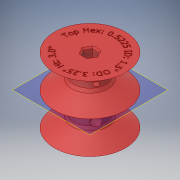
# Autodesk Inventor part: spoolV07
Saved by Autodesk Inventor 2019.4 (Build 234330000, 330)
## iProperties
Created: 2019-02-25
Part Number: spoolV07
Material: PC/ABS Plastic
Document SubType Name: Modeling
Designer: steele
Density: 0.357273 g/cm^3
Appearance: Smooth - Red
holeForString: 0.200 in
stringDiameter: 0.120 in
clearanceForString: 0.080 in
clearanceForHexShaft: 0.023 in
hexDiameter: 0.523 in
supportChannels: 0.150 in
spoolInteriorDiameter: 1.500 in
spoolInteriroRadius: 0.750 in
spoolExteriorDiameter: 3.250 in
spoolExteriorRadius: 1.625 in
spoolFiletRadius: 0.075 in
holeCenter: 0.575 in
hexHoleChamfer: 0.063 in
stringHoleCenterFromHexShaft: 0.361 in
textCircleDiameter: 2.438 in
textHeight: 0.240 in
textDepth: 0.050 in
stringHoleChamfer: 0.188 in
spoolTotalHeight: 3.000 in
spaceHeight: 0.250 in
spacerDiameter: 0.950 in
spoolHeightWithoutSpacer: 2.750 in
Author: steele
Autodesk Inventor part; units mm, degrees
(part 1 of 2)
ref_plane "XZ Plane" through (0, 0, 0) normal (0, 1, 0) x (-1, 0, 0)
ref_plane "XY Plane" through (0, 0, 0) normal (0, 0, 1) x (1, 0, 0)
sketch "Sketch15" plane through (0, 0, 0) normal (0, 0, 1) x (1, 0, 0)
  line L0 (41.275, 0) -> (41.275, 76.2) construction
  line L1 (0, 0) -> (41.275, 0)
  line L2 (0, 76.2) -> (41.275, 76.2)
  line L3 (19.05, 0) -> (19.05, 76.2) construction
  line L4 (0, 76.2) -> (0, 0)
  line L5 (19.05, 19.05) -> (41.275, 19.05) construction
  line L6 (41.275, 0) -> (19.05, 12.8316)
  line L7 (41.275, 38.1) -> (19.05, 25.2684)
  line L8 (19.05, 25.2684) -> (41.275, 25.2684) construction
  line L9 (19.05, 25.2684) -> (19.05, 12.8316)
  line L10 (41.275, 38.1) -> (19.05, 50.9316)
  line L11 (19.05, 50.9316) -> (19.05, 63.3684)
  line L12 (19.05, 63.3684) -> (41.275, 76.2)
  line L13 (41.275, 38.1) -> (19.05, 38.1) construction
  line L14 (19.05, 63.3684) -> (41.275, 63.3684) construction
  dimension "d85" = 41.275
  dimension "d86" = 76.2
  dimension "d87" = 19.05
  dimension "d88" = 41.275
  dimension "d89" = 38.1
  dimension "centerLineForSpool" = 19.05
  dimension "d93" = 30
  dimension "d94" = 30
  dimension "d95" = 30
  dimension "d96" = 30
  constraints: 30 end point, 10 point on line, 3 horizontal, 2 midpoint, 2 perpendicular, 1 collinear, 1 parallel, 1 vertical
  measures "d85" distance from line of L1.start L0
  measures "d86" distance of L0.start L0.end
  measures "d87" distance from line of L3 L1.start
  measures "d88" distance of L2.start L0.end
  measures "d89" distance from line of L7.start L1
  measures "centerLineForSpool" distance from line of L5.start L1
  measures "d93" angle of L6 L1
  measures "d94" angle of L7 L8
  measures "d95" angle of L10 L13
  measures "d96" angle of L12 L14
revolve "Revolution2" add sketch "Sketch15" angle 360 about axis through (0, 76.2, 0) along (0, -1, 0)
sketch "Sketch16" plane through (0, 0, 0) normal (0, -1, 0) x (1, 0, 0)
  line L0 (-7.6623, 0) -> (-3.8312, 6.6357)
  line L1 (-3.8312, 6.6357) -> (3.8312, 6.6357)
  line L2 (3.8312, 6.6357) -> (7.6623, 0)
  line L3 (7.6623, 0) -> (3.8312, -6.6358)
  line L4 (3.8312, -6.6358) -> (-3.8312, -6.6358)
  line L5 (-3.8312, -6.6358) -> (-7.6623, 0)
  point P0 (0, 0)
  point P1 (0, 0)
  dimension "d103" = 13.2715
  constraints: 12 end point, 1 coincident, 1 horizontal, 13 other
  measures "d103" distance between parallel lines of L1 L4
extrude "Extrusion11" cut sketch "Sketch16" against normal through all
sketch "Sketch17" plane through (0, 0, 0) normal (1, 0, 0) x (0, 1, 0)
  circle A0 centre (57.15, 9.1757) radius 2.54
  circle A1 centre (19.05, 9.1757) radius 2.54
  line L0 (0, 41.275) -> (0, -41.275) projected
  line L1 (76.2, 41.275) -> (76.2, -41.275) projected
  line L2 (0, 6.6357) -> (76.2, 6.6357) projected
  point P0 (0, 0)
  dimension "d110" = 19.05
  dimension "d111" = 19.05
  dimension "d112" = 5.08
  constraints: 2 centre point, 2 tangent, 1 equal radius
  measures "d110" distance from line of A1.centre L0
  measures "d111" distance from line of A0.centre L1
  measures "d112" diameter of A0
extrude "Extrusion13" cut sketch "Sketch17" along normal through all both and the other way through all
ref_plane "Work Plane4" through (-19.05, 0, 0) normal (1, 0, 0) x (0, 1, 0)
sketch "Sketch22" plane through (-19.05, 0, 0) normal (1, 0, 0) x (0, 1, 0)
  spline S0 degree 8 poles (59.69, 9.1757) (59.69, 9.4517) (59.6557, 9.7212) (59.59, 9.9804) (59.4956, 10.2261) (59.3755, 10.4557) (59.2323, 10.6669) (59.0691, 10.858) (58.7144, 11.191) (58.5225, 11.336) (58.3154, 11.4599) (58.0958, 11.5609) (57.8667, 11.6378) (57.6308, 11.6896) (57.3909, 11.7157) (56.8686, 11.7157) (56.5893, 11.6801) (56.3163, 11.6098) (56.0539, 11.5059) (55.8062, 11.37) (55.5775, 11.2041) (55.3719, 11.0111) (55.0147, 10.5794) (54.8595, 10.3366) (54.7333, 10.0693) (54.6415, 9.7817) (54.5882, 9.479) (54.5771, 9.1672) (54.6105, 8.8531) (54.8032, 8.1024) (55.0034, 7.6991) (55.2751, 7.3483) (55.6037, 7.0608) (55.9729, 6.8444) (56.3656, 6.703) (56.7635, 6.6357) (57.4276, 6.6357) (57.7065, 6.6704) (57.9827, 6.7403) (58.2517, 6.8459) (58.509, 6.9871) (58.7494, 7.1637) (58.9676, 7.3748) (59.2832, 7.7816) (59.3962, 7.9584) (59.4932, 8.1474) (59.5721, 8.3459) (59.6315, 8.5511) (59.6708, 8.76) (59.69, 8.9692) (59.69, 9.1757) knots 0 0 0 0 0 0 0 0 0 0.129052 0.129052 0.129052 0.129052 0.129052 0.129052 0.129052 0.253777 0.253777 0.253777 0.253777 0.253777 0.253777 0.253777 0.399469 0.399469 0.399469 0.399469 0.399469 0.399469 0.399469 0.544533 0.544533 0.544533 0.544533 0.544533 0.544533 0.544533 0.751894 0.751894 0.751894 0.751894 0.751894 0.751894 0.751894 0.900801 0.900801 0.900801 0.900801 0.900801 0.900801 0.900801 1 1 1 1 1 1 1 1 1 projected
  circle A0 centre (57.15, 9.1757) radius 4.7625
  circle A1 centre (57.15, 9.1757) radius 2.54 construction
  line L0 (57.15, 6.6357) -> (76.2, 6.6357) construction
  line L1 (76.2, 41.275) -> (76.2, -41.275) construction
  point P0 (0, 0)
  dimension "d121" = 19.05
  dimension "d122" = 5.08
  dimension "d125" = 9.525
  constraints: 2 centre point, 1 concentric, 1 tangent, 1 vertical alignment
  measures "d121" distance from line of A1.centre L1
  measures "d122" diameter of A1
  measures "d125" diameter of A0
extrude "Extrusion16" cut sketch "Sketch22" along normal blind 11.1125
ref_plane "Work Plane5" through (19.05, 0, 0) normal (1, 0, 0) x (0, 1, 0)
sketch "Sketch23" plane through (19.05, 0, 0) normal (1, 0, 0) x (0, 1, 0)
  line L0 (19.05, 6.6357) -> (57.15, 6.6357) projected
  circle A0 centre (19.05, 9.1757) radius 2.54 construction
  line L1 (0, 41.275) -> (0, -41.275) projected
  circle A1 centre (19.05, 9.1757) radius 4.7625
  point P0 (0, 0)
  dimension "d127" = 5.08
  dimension "d128" = 19.05
  dimension "d129" = 9.525
  constraints: 2 centre point, 1 coincident, 1 tangent
  measures "d127" diameter of A0
  measures "d128" distance from line of A0.centre L1
  measures "d129" diameter of A1
extrude "Extrusion17" cut sketch "Sketch23" against normal blind 11.1125
chamfer "Chamfer10" distance 1.5875 angle 45 12 edges at (0, 76.2, -6.6358) (5.7467, 76.2, -3.3179) (5.7467, 76.2, 3.3179) (0, 76.2, 6.6357) (-5.7467, 76.2, 3.3179) (-5.7467, 76.2, -3.3179) (-5.7467, 0, -3.3179) (-5.7467, 0, 3.3179) (0, 0, 6.6357) (5.7467, 0, 3.3179) (5.7467, 0, -3.3179) (0, 0, -6.6358)
chamfer "Chamfer12" distance 2.3813 angle 45 4 edges at (-19.05, 63.3684, 0) (-19.05, 50.9316, 0) (-19.05, 25.2684, 0) (-19.05, 12.8316, 0)
ref_plane "Work Plane6" through (0, 38.1, 0) normal (0, -1, 0) x (1, 0, 0)
sketch "Sketch24" plane through (0, 76.2, 0) normal (0, 1, 0) x (1, 0, 0)
  circle A0 centre (0, 0) radius 28.575 construction
  line L0 (-28.5056, 2.0328) -> (-33.8607, 2.492)
  line L1 (-33.8607, 2.492) -> (-34.0354, 0.4543)
  line L2 (-34.0354, 0.4543) -> (-34.754, 0.5159)
  line L3 (-34.754, 0.5159) -> (-34.3353, 5.3985)
  line L4 (-34.3353, 5.3985) -> (-33.6167, 5.3369)
  line L5 (-33.6167, 5.3369) -> (-33.7914, 3.2992)
  line L6 (-33.7914, 3.2992) -> (-28.4363, 2.84)
  line L7 (-28.4363, 2.84) -> (-28.5056, 2.0328)
  spline S0 degree 2 poles (-29.3924, 9.63) (-28.2725, 9.3434) (-27.3277, 7.9543) (-27.5579, 7.0546) knots 0 0 0 1 2 2 2
  spline S1 degree 2 poles (-27.5579, 7.0546) (-27.7943, 6.1309) (-29.3236, 5.3953) (-30.4052, 5.6721) knots 0 0 0 1 2 2 2
  spline S2 degree 2 poles (-30.4052, 5.6721) (-31.5155, 5.9562) (-32.4663, 7.3621) (-32.2385, 8.2523) knots 0 0 0 1 2 2 2
  spline S3 degree 2 poles (-32.2385, 8.2523) (-32.0082, 9.152) (-30.5075, 9.9153) (-29.3924, 9.63) knots 0 0 0 1 2 2 2
  spline S4 degree 2 poles (-29.5896, 8.8595) (-30.451, 9.0799) (-31.449, 8.6673) (-31.5972, 8.0882) knots 0 0 0 1 2 2 2
  spline S5 degree 2 poles (-31.5972, 8.0882) (-31.7454, 7.5091) (-31.0695, 6.6631) (-30.208, 6.4426) knots 0 0 0 1 2 2 2
  spline S6 degree 2 poles (-30.208, 6.4426) (-29.3705, 6.2283) (-28.3474, 6.6396) (-28.1992, 7.2187) knots 0 0 0 1 2 2 2
  spline S7 degree 2 poles (-28.1992, 7.2187) (-28.0523, 7.793) (-28.7377, 8.6415) (-29.5896, 8.8595) knots 0 0 0 1 2 2 2
  spline S8 degree 2 poles (-27.5782, 14.278) (-26.5275, 13.8203) (-25.7227, 12.2788) (-26.0561, 11.5134) knots 0 0 0 1 2 2 2
  spline S9 degree 2 poles (-26.0561, 11.5134) (-26.1923, 11.2009) (-26.5463, 10.784) (-26.8043, 10.6) knots 0 0 0 1 2 2 2
  line L8 (-26.8043, 10.6) -> (-25.0471, 9.8344)
  line L9 (-25.0471, 9.8344) -> (-25.3549, 9.1279)
  line L10 (-25.3549, 9.1279) -> (-31.093, 11.6278)
  line L11 (-31.093, 11.6278) -> (-30.7852, 12.3343)
  line L12 (-30.7852, 12.3343) -> (-30.3459, 12.1429)
  spline S10 degree 2 poles (-30.3459, 12.1429) (-30.4715, 12.5102) (-30.5083, 13.2914) (-30.3446, 13.6673) knots 0 0 0 1 2 2 2
  spline S11 degree 2 poles (-30.3446, 13.6673) (-30.0308, 14.3874) (-28.5384, 14.6963) (-27.5782, 14.278) knots 0 0 0 1 2 2 2
  spline S12 degree 2 poles (-27.8144, 13.5133) (-28.5345, 13.8271) (-29.5263, 13.7149) (-29.7493, 13.2032) knots 0 0 0 1 2 2 2
  spline S13 degree 2 poles (-29.7493, 13.2032) (-29.8795, 12.9043) (-29.8569, 12.2263) (-29.7571, 11.8864) knots 0 0 0 1 2 2 2
  line L13 (-29.7571, 11.8864) -> (-27.3749, 10.8486)
  spline S14 degree 2 poles (-27.3749, 10.8486) (-27.1232, 11.0676) (-26.852, 11.4182) (-26.7415, 11.6718) knots 0 0 0 1 2 2 2
  spline S15 degree 2 poles (-26.7415, 11.6718) (-26.5027, 12.2198) (-27.0445, 13.1779) (-27.8144, 13.5133) knots 0 0 0 1 2 2 2
  line L14 (-20.7867, 19.7317) -> (-21.2974, 19.1028)
  line L15 (-21.2974, 19.1028) -> (-23.6136, 20.9838)
  line L16 (-23.6136, 20.9838) -> (-25.3825, 18.8057)
  line L17 (-25.3825, 18.8057) -> (-23.0663, 16.9247)
  line L18 (-23.0663, 16.9247) -> (-23.577, 16.2958)
  line L19 (-23.577, 16.2958) -> (-28.3092, 20.1387)
  line L20 (-28.3092, 20.1387) -> (-27.7984, 20.7676)
  line L21 (-27.7984, 20.7676) -> (-25.9424, 19.2603)
  line L22 (-25.9424, 19.2603) -> (-24.1735, 21.4385)
  line L23 (-24.1735, 21.4385) -> (-26.0296, 22.9458)
  line L24 (-26.0296, 22.9458) -> (-25.5188, 23.5747)
  line L25 (-25.5188, 23.5747) -> (-20.7867, 19.7317)
  spline S16 degree 2 poles (-18.3661, 21.758) (-19.1957, 21.0407) (-20.912, 21.1828) (-21.6552, 22.0423) knots 0 0 0 1 2 2 2
  spline S17 degree 2 poles (-21.6552, 22.0423) (-22.3854, 22.8868) (-22.3657, 24.654) (-21.652, 25.2712) knots 0 0 0 1 2 2 2
  spline S18 degree 2 poles (-21.652, 25.2712) (-21.3306, 25.5491) (-20.6721, 25.792) (-20.3177, 25.7522) knots 0 0 0 1 2 2 2
  spline S19 degree 2 poles (-20.3177, 25.7522) (-19.9596, 25.7157) (-19.2672, 25.3152) (-18.9086, 24.9005) knots 0 0 0 1 2 2 2
  line L26 (-18.9086, 24.9005) -> (-18.6339, 24.5828)
  line L27 (-18.6339, 24.5828) -> (-21.0292, 22.5117)
  spline S20 degree 2 poles (-21.0292, 22.5117) (-20.509, 21.9101) (-19.3511, 21.7945) (-18.813, 22.2598) knots 0 0 0 1 2 2 2
  spline S21 degree 2 poles (-18.813, 22.2598) (-18.6225, 22.4246) (-18.3268, 22.8304) (-18.2355, 23.0269) knots 0 0 0 1 2 2 2
  spline S22 degree 2 poles (-18.2355, 23.0269) (-18.1432, 23.2373) (-18.0396, 23.5555) (-18.0203, 23.6767) knots 0 0 0 1 2 2 2
  line L28 (-18.0203, 23.6767) -> (-17.9866, 23.7058)
  line L29 (-17.9866, 23.7058) -> (-17.4373, 23.0705)
  spline S23 degree 2 poles (-17.4373, 23.0705) (-17.5027, 22.9422) (-17.7057, 22.5577) (-17.7962, 22.4206) knots 0 0 0 1 2 2 2
  spline S24 degree 2 poles (-17.7962, 22.4206) (-17.9224, 22.2267) (-18.1569, 21.939) (-18.3661, 21.758) knots 0 0 0 1 2 2 2
  spline S25 degree 2 poles (-19.5864, 24.5364) (-19.7975, 24.7653) (-20.1919, 25.0251) (-20.3855, 25.0602) knots 0 0 0 1 2 2 2
  spline S26 degree 2 poles (-20.3855, 25.0602) (-20.5995, 25.1037) (-21.0366, 24.9673) (-21.2721, 24.7638) knots 0 0 0 1 2 2 2
  spline S27 degree 2 poles (-21.2721, 24.7638) (-21.5037, 24.5635) (-21.7093, 24.1441) (-21.7275, 23.8932) knots 0 0 0 1 2 2 2
  spline S28 degree 2 poles (-21.7275, 23.8932) (-21.7387, 23.6419) (-21.5857, 23.193) (-21.4137, 22.9564) knots 0 0 0 1 2 2 2
  line L30 (-21.4137, 22.9564) -> (-19.5864, 24.5364)
  line L31 (-13.5409, 25.2452) -> (-14.3386, 24.7412)
  line L32 (-14.3386, 24.7412) -> (-16.1964, 25.601)
  line L33 (-16.1964, 25.601) -> (-16.243, 23.5381)
  line L34 (-16.243, 23.5381) -> (-16.9823, 23.0711)
  line L35 (-16.9823, 23.0711) -> (-16.8526, 25.835)
  line L36 (-16.8526, 25.835) -> (-19.4129, 26.9464)
  line L37 (-19.4129, 26.9464) -> (-18.6152, 27.4503)
  line L38 (-18.6152, 27.4503) -> (-16.7694, 26.6005)
  line L39 (-16.7694, 26.6005) -> (-16.7233, 28.6455)
  line L40 (-16.7233, 28.6455) -> (-15.984, 29.1125)
  line L41 (-15.984, 29.1125) -> (-16.1106, 26.3623)
  line L42 (-16.1106, 26.3623) -> (-13.5409, 25.2452)
  line L43 (-13.1552, 29.157) -> (-14.0405, 28.7412)
  line L44 (-14.0405, 28.7412) -> (-14.5362, 29.7964)
  line L45 (-14.5362, 29.7964) -> (-13.6509, 30.2123)
  line L46 (-13.6509, 30.2123) -> (-13.1552, 29.157)
  line L47 (-11.706, 26.0718) -> (-12.5914, 25.6559)
  line L48 (-12.5914, 25.6559) -> (-13.087, 26.7112)
  line L49 (-13.087, 26.7112) -> (-12.2017, 27.127)
  line L50 (-12.2017, 27.127) -> (-11.706, 26.0718)
  spline S29 degree 2 poles (-4.8677, 31.307) (-4.5164, 29.705) (-5.1186, 28) (-6.0885, 27.7873) knots 0 0 0 1 2 2 2
  spline S30 degree 2 poles (-6.0885, 27.7873) (-7.0729, 27.5715) (-8.33, 28.899) (-8.6739, 30.4673) knots 0 0 0 1 2 2 2
  spline S31 degree 2 poles (-8.6739, 30.4673) (-9.0273, 32.0789) (-8.423, 33.7742) (-7.4483, 33.9879) knots 0 0 0 1 2 2 2
  spline S32 degree 2 poles (-7.4483, 33.9879) (-6.4687, 34.2028) (-5.2085, 32.8607) (-4.8677, 31.307) knots 0 0 0 1 2 2 2
  spline S33 degree 2 poles (-5.4928, 29.2683) (-5.4416, 29.5881) (-5.544, 30.5164) (-5.6784, 31.1292) knots 0 0 0 1 2 2 2
  spline S34 degree 2 poles (-5.6784, 31.1292) (-5.8128, 31.742) (-6.1072, 32.6232) (-6.2945, 32.9008) knots 0 0 0 1 2 2 2
  spline S35 degree 2 poles (-6.2945, 32.9008) (-6.4818, 33.1783) (-6.9704, 33.3999) (-7.3033, 33.3269) knots 0 0 0 1 2 2 2
  spline S36 degree 2 poles (-7.3033, 33.3269) (-7.6363, 33.2539) (-7.9969, 32.846) (-8.0536, 32.5049) knots 0 0 0 1 2 2 2
  spline S37 degree 2 poles (-8.0536, 32.5049) (-8.1076, 32.1744) (-7.9913, 31.2289) (-7.8632, 30.645) knots 0 0 0 1 2 2 2
  spline S38 degree 2 poles (-7.8632, 30.645) (-7.7257, 30.0177) (-7.4643, 29.195) (-7.2669, 28.8944) knots 0 0 0 1 2 2 2
  spline S39 degree 2 poles (-7.2669, 28.8944) (-7.0834, 28.611) (-6.5809, 28.3722) (-6.2335, 28.4484) knots 0 0 0 1 2 2 2
  spline S40 degree 2 poles (-6.2335, 28.4484) (-5.9054, 28.5204) (-5.5447, 28.9282) (-5.4928, 29.2683) knots 0 0 0 1 2 2 2
  line L51 (-2.1318, 28.4995) -> (-3.1058, 28.41)
  line L52 (-3.1058, 28.41) -> (-3.2125, 29.571)
  line L53 (-3.2125, 29.571) -> (-2.2384, 29.6604)
  line L54 (-2.2384, 29.6604) -> (-2.1318, 28.4995)
  spline S41 degree 2 poles (2.8482, 30.4347) (2.8338, 29.9953) (2.5279, 29.254) (2.2621, 28.9859) knots 0 0 0 1 2 2 2
  spline S42 degree 2 poles (2.2621, 28.9859) (1.9963, 28.7178) (1.2205, 28.4219) (0.7465, 28.4373) knots 0 0 0 1 2 2 2
  spline S43 degree 2 poles (0.7465, 28.4373) (0.312, 28.4515) (-0.5309, 28.6719) (-0.8369, 28.8351) knots 0 0 0 1 2 2 2
  line L55 (-0.8369, 28.8351) -> (-0.8087, 29.6991)
  line L56 (-0.8087, 29.6991) -> (-0.7495, 29.6972)
  spline S44 degree 2 poles (-0.7495, 29.6972) (-0.6579, 29.625) (-0.3132, 29.4358) (-0.1034, 29.3499) knots 0 0 0 1 2 2 2
  spline S45 degree 2 poles (-0.1034, 29.3499) (0.1358, 29.258) (0.5326, 29.1511) (0.7844, 29.1429) knots 0 0 0 1 2 2 2
  spline S46 degree 2 poles (0.7844, 29.1429) (1.0313, 29.1348) (1.5012, 29.2974) (1.6754, 29.4845) knots 0 0 0 1 2 2 2
  spline S47 degree 2 poles (1.6754, 29.4845) (1.8344, 29.6622) (2.0082, 30.1409) (2.0189, 30.4667) knots 0 0 0 1 2 2 2
  spline S48 degree 2 poles (2.0189, 30.4667) (2.0295, 30.7926) (1.8653, 31.2132) (1.702, 31.3569) knots 0 0 0 1 2 2 2
  spline S49 degree 2 poles (1.702, 31.3569) (1.5342, 31.5156) (1.0249, 31.6608) (0.7138, 31.6709) knots 0 0 0 1 2 2 2
  spline S50 degree 2 poles (0.7138, 31.6709) (0.3781, 31.6819) (-0.2919, 31.6) (-0.4957, 31.5622) knots 0 0 0 1 2 2 2
  line L57 (-0.4957, 31.5622) -> (-0.3931, 34.7024)
  line L58 (-0.3931, 34.7024) -> (2.9495, 34.5931)
  line L59 (2.9495, 34.5931) -> (2.9261, 33.8772)
  line L60 (2.9261, 33.8772) -> (0.3685, 33.9608)
  line L61 (0.3685, 33.9608) -> (0.3154, 32.3364)
  spline S51 degree 2 poles (0.3154, 32.3364) (0.4642, 32.3513) (0.7511, 32.3567) (0.8696, 32.3529) knots 0 0 0 1 2 2 2
  spline S52 degree 2 poles (0.8696, 32.3529) (1.3386, 32.3375) (1.9804, 32.1633) (2.2692, 31.9265) knots 0 0 0 1 2 2 2
  spline S53 degree 2 poles (2.2692, 31.9265) (2.563, 31.6896) (2.8663, 30.9877) (2.8482, 30.4347) knots 0 0 0 1 2 2 2
  line L62 (7.3458, 27.6811) -> (3.6558, 28.4)
  line L63 (3.6558, 28.4) -> (3.8211, 29.2486)
  spline S54 degree 2 poles (3.8211, 29.2486) (4.2915, 29.5445) (5.1345, 30.0999) (5.5467, 30.4072) knots 0 0 0 1 2 2 2
  spline S55 degree 2 poles (5.5467, 30.4072) (6.3768, 31.0255) (7.0519, 31.8301) (7.1455, 32.3102) knots 0 0 0 1 2 2 2
  spline S56 degree 2 poles (7.1455, 32.3102) (7.1946, 32.5623) (7.1131, 32.9707) (6.9961, 33.1194) knots 0 0 0 1 2 2 2
  spline S57 degree 2 poles (6.9961, 33.1194) (6.8791, 33.268) (6.5342, 33.461) (6.3112, 33.5044) knots 0 0 0 1 2 2 2
  spline S58 degree 2 poles (6.3112, 33.5044) (6.0978, 33.546) (5.6406, 33.5244) (5.4258, 33.4807) knots 0 0 0 1 2 2 2
  spline S59 degree 2 poles (5.4258, 33.4807) (5.2428, 33.4458) (4.8899, 33.3133) (4.7797, 33.2643) knots 0 0 0 1 2 2 2
  line L64 (4.7797, 33.2643) -> (4.736, 33.2728)
  line L65 (4.736, 33.2728) -> (4.9023, 34.1262)
  spline S60 degree 2 poles (4.9023, 34.1262) (5.1732, 34.1992) (6.1068, 34.264) (6.5044, 34.1865) knots 0 0 0 1 2 2 2
  spline S61 degree 2 poles (6.5044, 34.1865) (7.3433, 34.0231) (8.116, 32.9515) (7.9686, 32.1951) knots 0 0 0 1 2 2 2
  spline S62 degree 2 poles (7.9686, 32.1951) (7.8996, 31.8411) (7.6195, 31.2817) (7.4249, 31.0579) knots 0 0 0 1 2 2 2
  spline S63 degree 2 poles (7.4249, 31.0579) (7.2284, 30.8244) (6.7064, 30.3926) (6.4255, 30.1906) knots 0 0 0 1 2 2 2
  spline S64 degree 2 poles (6.4255, 30.1906) (5.967, 29.8522) (4.8689, 29.1501) (4.5425, 28.947) knots 0 0 0 1 2 2 2
  line L66 (4.5425, 28.947) -> (7.4809, 28.3745)
  line L67 (7.4809, 28.3745) -> (7.3458, 27.6811)
  line L68 (11.6554, 26.1602) -> (8.1268, 27.4569)
  line L69 (8.1268, 27.4569) -> (8.425, 28.2683)
  spline S65 degree 2 poles (8.425, 28.2683) (8.9364, 28.4857) (9.8571, 28.9) (10.3128, 29.1377) knots 0 0 0 1 2 2 2
  spline S66 degree 2 poles (10.3128, 29.1377) (11.2308, 29.6162) (12.0253, 30.3031) (12.194, 30.7622) knots 0 0 0 1 2 2 2
  spline S67 degree 2 poles (12.194, 30.7622) (12.2826, 31.0033) (12.2671, 31.4195) (12.1752, 31.5848) knots 0 0 0 1 2 2 2
  spline S68 degree 2 poles (12.1752, 31.5848) (12.0834, 31.7502) (11.7736, 31.9956) (11.5603, 32.074) knots 0 0 0 1 2 2 2
  spline S69 degree 2 poles (11.5603, 32.074) (11.3563, 32.1489) (10.9015, 32.2003) (10.6824, 32.1913) knots 0 0 0 1 2 2 2
  spline S70 degree 2 poles (10.6824, 32.1913) (10.4962, 32.186) (10.1267, 32.1113) (10.0101, 32.0805) knots 0 0 0 1 2 2 2
  line L70 (10.0101, 32.0805) -> (9.9683, 32.0958)
  line L71 (9.9683, 32.0958) -> (10.2682, 32.9119)
  spline S71 degree 2 poles (10.2682, 32.9119) (10.5473, 32.9409) (11.4794, 32.8563) (11.8596, 32.7166) knots 0 0 0 1 2 2 2
  spline S72 degree 2 poles (11.8596, 32.7166) (12.6618, 32.4218) (13.2541, 31.241) (12.9883, 30.5176) knots 0 0 0 1 2 2 2
  spline S73 degree 2 poles (12.9883, 30.5176) (12.8639, 30.1791) (12.4984, 29.6714) (12.2707, 29.4814) knots 0 0 0 1 2 2 2
  spline S74 degree 2 poles (12.2707, 29.4814) (12.0396, 29.2821) (11.4555, 28.9388) (11.1461, 28.7842) knots 0 0 0 1 2 2 2
  spline S75 degree 2 poles (11.1461, 28.7842) (10.6395, 28.5229) (9.4438, 28.0045) (9.0892, 27.8559) knots 0 0 0 1 2 2 2
  line L72 (9.0892, 27.8559) -> (11.8991, 26.8233)
  line L73 (11.8991, 26.8233) -> (11.6554, 26.1602)
  spline S76 degree 2 poles (16.5609, 25.6928) (16.3455, 25.3095) (15.7322, 24.7928) (15.3727, 24.6775) knots 0 0 0 1 2 2 2
  spline S77 degree 2 poles (15.3727, 24.6775) (15.0133, 24.5621) (14.1884, 24.6573) (13.775, 24.8896) knots 0 0 0 1 2 2 2
  spline S78 degree 2 poles (13.775, 24.8896) (13.396, 25.1025) (12.7496, 25.6867) (12.5533, 25.9726) knots 0 0 0 1 2 2 2
  line L74 (12.5533, 25.9726) -> (12.9767, 26.7263)
  line L75 (12.9767, 26.7263) -> (13.0284, 26.6973)
  spline S79 degree 2 poles (13.0284, 26.6973) (13.0764, 26.591) (13.295, 26.2642) (13.4415, 26.0912) knots 0 0 0 1 2 2 2
  spline S80 degree 2 poles (13.4415, 26.0912) (13.6114, 25.8994) (13.9143, 25.6216) (14.1339, 25.4982) knots 0 0 0 1 2 2 2
  spline S81 degree 2 poles (14.1339, 25.4982) (14.3493, 25.3772) (14.8412, 25.3048) (15.082, 25.3904) knots 0 0 0 1 2 2 2
  spline S82 degree 2 poles (15.082, 25.3904) (15.3051, 25.4748) (15.68, 25.8194) (15.8397, 26.1037) knots 0 0 0 1 2 2 2
  spline S83 degree 2 poles (15.8397, 26.1037) (15.9994, 26.3879) (16.0477, 26.8368) (15.969, 27.0397) knots 0 0 0 1 2 2 2
  spline S84 degree 2 poles (15.969, 27.0397) (15.8933, 27.2579) (15.5083, 27.6215) (15.237, 27.7739) knots 0 0 0 1 2 2 2
  spline S85 degree 2 poles (15.237, 27.7739) (14.9441, 27.9385) (14.3119, 28.1747) (14.1135, 28.2352) knots 0 0 0 1 2 2 2
  line L76 (14.1135, 28.2352) -> (15.6525, 30.9743)
  line L77 (15.6525, 30.9743) -> (18.5682, 29.3361)
  line L78 (18.5682, 29.3361) -> (18.2173, 28.7116)
  line L79 (18.2173, 28.7116) -> (15.9864, 29.9651)
  line L80 (15.9864, 29.9651) -> (15.1903, 28.5481)
  spline S86 degree 2 poles (15.1903, 28.5481) (15.3292, 28.4928) (15.5862, 28.3653) (15.6896, 28.3073) knots 0 0 0 1 2 2 2
  spline S87 degree 2 poles (15.6896, 28.3073) (16.0987, 28.0774) (16.5879, 27.6269) (16.735, 27.2836) knots 0 0 0 1 2 2 2
  spline S88 degree 2 poles (16.735, 27.2836) (16.8864, 26.9378) (16.8319, 26.1752) (16.5609, 25.6928) knots 0 0 0 1 2 2 2
  line L81 (20.0973, 20.3474) -> (18.3504, 21.9362)
  line L82 (18.3504, 21.9362) -> (18.7691, 22.3966)
  line L83 (18.7691, 22.3966) -> (19.3429, 21.8748)
  line L84 (19.3429, 21.8748) -> (22.6068, 25.4637)
  line L85 (22.6068, 25.4637) -> (22.033, 25.9856)
  line L86 (22.033, 25.9856) -> (22.4518, 26.446)
  line L87 (22.4518, 26.446) -> (24.1988, 24.8573)
  line L88 (24.1988, 24.8573) -> (23.78, 24.3968)
  line L89 (23.78, 24.3968) -> (23.2062, 24.9186)
  line L90 (23.2062, 24.9186) -> (19.9423, 21.3297)
  line L91 (19.9423, 21.3297) -> (20.5161, 20.8079)
  line L92 (20.5161, 20.8079) -> (20.0973, 20.3474)
  spline S89 degree 2 poles (26.2269, 17.847) (25.5772, 17.3227) (24.1065, 17.0056) (23.4575, 17.2119) knots 0 0 0 1 2 2 2
  spline S90 degree 2 poles (23.4575, 17.2119) (22.9391, 17.3903) (22.1866, 18.0081) (21.7212, 18.5848) knots 0 0 0 1 2 2 2
  line L93 (21.7212, 18.5848) -> (20.8402, 19.6766)
  line L94 (20.8402, 19.6766) -> (25.5842, 23.5048)
  line L95 (25.5842, 23.5048) -> (26.456, 22.4245)
  spline S91 degree 2 poles (26.456, 22.4245) (26.9958, 21.7556) (27.4101, 20.8331) (27.4504, 20.4213) knots 0 0 0 1 2 2 2
  spline S92 degree 2 poles (27.4504, 20.4213) (27.5159, 19.7187) (26.9189, 18.4054) (26.2269, 17.847) knots 0 0 0 1 2 2 2
  spline S93 degree 2 poles (25.7041, 18.5106) (26.25, 18.9511) (26.7311, 19.936) (26.6617, 20.4704) knots 0 0 0 1 2 2 2
  spline S94 degree 2 poles (26.6617, 20.4704) (26.6069, 20.8451) (26.2792, 21.5265) (25.9349, 21.9533) knots 0 0 0 1 2 2 2
  line L96 (25.9349, 21.9533) -> (25.5471, 22.4338)
  line L97 (25.5471, 22.4338) -> (21.8949, 19.4867)
  line L98 (21.8949, 19.4867) -> (22.2827, 19.0061)
  spline S95 degree 2 poles (22.2827, 19.0061) (22.6208, 18.5871) (23.2672, 18.0613) (23.6558, 17.9495) knots 0 0 0 1 2 2 2
  spline S96 degree 2 poles (23.6558, 17.9495) (24.1456, 17.7988) (25.1505, 18.0639) (25.7041, 18.5106) knots 0 0 0 1 2 2 2
  line L99 (24.9302, 13.9733) -> (24.4375, 14.8182)
  line L100 (24.4375, 14.8182) -> (25.4446, 15.4056)
  line L101 (25.4446, 15.4056) -> (25.9373, 14.5607)
  line L102 (25.9373, 14.5607) -> (24.9302, 13.9733)
  line L103 (27.8747, 15.6905) -> (27.3819, 16.5355)
  line L104 (27.3819, 16.5355) -> (28.389, 17.1228)
  line L105 (28.389, 17.1228) -> (28.8818, 16.2779)
  line L106 (28.8818, 16.2779) -> (27.8747, 15.6905)
  line L107 (27.7417, 7.0372) -> (26.8494, 9.8741)
  line L108 (26.8494, 9.8741) -> (27.4432, 10.0608)
  line L109 (27.4432, 10.0608) -> (27.7752, 9.0052)
  line L110 (27.7752, 9.0052) -> (31.6724, 10.231)
  line L111 (31.6724, 10.231) -> (31.3404, 11.2866)
  line L112 (31.3404, 11.2866) -> (31.8729, 11.4541)
  spline S97 degree 2 poles (31.8729, 11.4541) (32.0611, 10.8556) (32.5783, 10.3968) (33.0614, 10.5073) knots 0 0 0 1 2 2 2
  line L113 (33.0614, 10.5073) -> (33.2511, 9.9041)
  line L114 (33.2511, 9.9041) -> (28.0109, 8.256)
  line L115 (28.0109, 8.256) -> (28.3355, 7.2239)
  line L116 (28.3355, 7.2239) -> (27.7417, 7.0372)
  line L117 (28.1979, 4.6523) -> (28.0223, 5.6145)
  line L118 (28.0223, 5.6145) -> (29.1693, 5.8237)
  line L119 (29.1693, 5.8237) -> (29.3448, 4.8615)
  line L120 (29.3448, 4.8615) -> (28.1979, 4.6523)
  spline S98 degree 2 poles (30.5674, -0.1364) (30.1284, -0.1611) (29.3629, 0.0779) (29.0723, 0.3189) knots 0 0 0 1 2 2 2
  spline S99 degree 2 poles (29.0723, 0.3189) (28.7816, 0.5598) (28.418, 1.3063) (28.3914, 1.7798) knots 0 0 0 1 2 2 2
  spline S100 degree 2 poles (28.3914, 1.7798) (28.367, 2.2138) (28.5117, 3.073) (28.6471, 3.3923) knots 0 0 0 1 2 2 2
  line L121 (28.6471, 3.3923) -> (29.5102, 3.4408)
  line L122 (29.5102, 3.4408) -> (29.5135, 3.3817)
  spline S101 degree 2 poles (29.5135, 3.3817) (29.4498, 3.2841) (29.2919, 2.9239) (29.2249, 2.7074) knots 0 0 0 1 2 2 2
  spline S102 degree 2 poles (29.2249, 2.7074) (29.1547, 2.461) (29.0834, 2.0562) (29.0976, 1.8046) knots 0 0 0 1 2 2 2
  spline S103 degree 2 poles (29.0976, 1.8046) (29.1114, 1.558) (29.3151, 1.1044) (29.5169, 0.9475) knots 0 0 0 1 2 2 2
  spline S104 degree 2 poles (29.5169, 0.9475) (29.7079, 0.8049) (30.2002, 0.6742) (30.5257, 0.6925) knots 0 0 0 1 2 2 2
  spline S105 degree 2 poles (30.5257, 0.6925) (30.8512, 0.7108) (31.2556, 0.9117) (31.3842, 1.0872) knots 0 0 0 1 2 2 2
  spline S106 degree 2 poles (31.3842, 1.0872) (31.5274, 1.2684) (31.6268, 1.7886) (31.6093, 2.0993) knots 0 0 0 1 2 2 2
  spline S107 degree 2 poles (31.6093, 2.0993) (31.5905, 2.4347) (31.4494, 3.0947) (31.3937, 3.2944) knots 0 0 0 1 2 2 2
  line L123 (31.3937, 3.2944) -> (34.5306, 3.4708)
  line L124 (34.5306, 3.4708) -> (34.7184, 0.1317)
  line L125 (34.7184, 0.1317) -> (34.0032, 0.0915)
  line L126 (34.0032, 0.0915) -> (33.8595, 2.6464)
  line L127 (33.8595, 2.6464) -> (32.2368, 2.5551)
  spline S108 degree 2 poles (32.2368, 2.5551) (32.2649, 2.4083) (32.2957, 2.123) (32.3024, 2.0047) knots 0 0 0 1 2 2 2
  spline S109 degree 2 poles (32.3024, 2.0047) (32.3288, 1.5361) (32.2122, 0.8814) (32.002, 0.5727) knots 0 0 0 1 2 2 2
  spline S110 degree 2 poles (32.002, 0.5727) (31.792, 0.2591) (31.1198, -0.1053) (30.5674, -0.1364) knots 0 0 0 1 2 2 2
  line L128 (34.8505, -2.5567) -> (32.502, -2.1841)
  line L129 (32.502, -2.1841) -> (32.5464, -1.6475)
  line L130 (32.5464, -1.6475) -> (34.9242, -1.6656)
  line L131 (34.9242, -1.6656) -> (34.8505, -2.5567)
  line L132 (34.7235, -4.0928) -> (32.375, -3.7201)
  line L133 (32.375, -3.7201) -> (32.4194, -3.1835)
  line L134 (32.4194, -3.1835) -> (34.7972, -3.2017)
  line L135 (34.7972, -3.2017) -> (34.7235, -4.0928)
  spline S111 degree 2 poles (31.4234, -13.0649) (30.9268, -13.2577) (29.6805, -13.2302) (28.9624, -12.9791) knots 0 0 0 1 2 2 2
  spline S112 degree 2 poles (28.9624, -12.9791) (28.2629, -12.7346) (27.2536, -11.9841) (26.9885, -11.5146) knots 0 0 0 1 2 2 2
  spline S113 degree 2 poles (26.9885, -11.5146) (26.7114, -11.02) (26.6567, -9.949) (26.8539, -9.3848) knots 0 0 0 1 2 2 2
  spline S114 degree 2 poles (26.8539, -9.3848) (27.0577, -8.8019) (27.7801, -8.0078) (28.2862, -7.8027) knots 0 0 0 1 2 2 2
  spline S115 degree 2 poles (28.2862, -7.8027) (28.7843, -7.6052) (30.032, -7.6437) (30.7409, -7.8915) knots 0 0 0 1 2 2 2
  spline S116 degree 2 poles (30.7409, -7.8915) (31.4637, -8.1441) (32.4387, -8.8879) (32.7193, -9.3576) knots 0 0 0 1 2 2 2
  spline S117 degree 2 poles (32.7193, -9.3576) (32.9844, -9.827) (33.0531, -10.9029) (32.8509, -11.4812) knots 0 0 0 1 2 2 2
  spline S118 degree 2 poles (32.8509, -11.4812) (32.6455, -12.0688) (31.9059, -12.8673) (31.4234, -13.0649) knots 0 0 0 1 2 2 2
  spline S119 degree 2 poles (29.2411, -12.1817) (29.81, -12.3806) (30.7778, -12.4415) (31.1452, -12.3188) knots 0 0 0 1 2 2 2
  spline S120 degree 2 poles (31.1452, -12.3188) (31.5235, -12.1946) (32.0469, -11.6554) (32.1871, -11.2544) knots 0 0 0 1 2 2 2
  spline S121 degree 2 poles (32.1871, -11.2544) (32.3322, -10.8393) (32.2615, -10.1134) (32.0369, -9.7679) knots 0 0 0 1 2 2 2
  spline S122 degree 2 poles (32.0369, -9.7679) (31.823, -9.4367) (31.0217, -8.8845) (30.4621, -8.6889) knots 0 0 0 1 2 2 2
  spline S123 degree 2 poles (30.4621, -8.6889) (29.3289, -8.2928) (27.7932, -8.8235) (27.5145, -9.6209) knots 0 0 0 1 2 2 2
  spline S124 degree 2 poles (27.5145, -9.6209) (27.2357, -10.4184) (28.1079, -11.7856) (29.2411, -12.1817) knots 0 0 0 1 2 2 2
  spline S125 degree 2 poles (25.8122, -18.4416) (25.0957, -18.0131) (24.2898, -16.7427) (24.2591, -16.0624) knots 0 0 0 1 2 2 2
  spline S126 degree 2 poles (24.2591, -16.0624) (24.2473, -15.5143) (24.5669, -14.5946) (24.9472, -13.9586) knots 0 0 0 1 2 2 2
  line L136 (24.9472, -13.9586) -> (25.6672, -12.7545)
  line L137 (25.6672, -12.7545) -> (30.8993, -15.8829)
  line L138 (30.8993, -15.8829) -> (30.1869, -17.0743)
  spline S127 degree 2 poles (30.1869, -17.0743) (29.7457, -17.8121) (29.0233, -18.5197) (28.6508, -18.6999) knots 0 0 0 1 2 2 2
  spline S128 degree 2 poles (28.6508, -18.6999) (28.0142, -19.0042) (26.5754, -18.8979) (25.8122, -18.4416) knots 0 0 0 1 2 2 2
  spline S129 degree 2 poles (26.2542, -17.7216) (26.8563, -18.0816) (27.9468, -18.1927) (28.4243, -17.9429) knots 0 0 0 1 2 2 2
  spline S130 degree 2 poles (28.4243, -17.9429) (28.757, -17.7619) (29.2831, -17.2189) (29.5645, -16.7483) knots 0 0 0 1 2 2 2
  line L139 (29.5645, -16.7483) -> (29.8814, -16.2183)
  line L140 (29.8814, -16.2183) -> (25.8535, -13.8098)
  line L141 (25.8535, -13.8098) -> (25.5366, -14.3398)
  spline S131 degree 2 poles (25.5366, -14.3398) (25.2603, -14.802) (24.9904, -15.5903) (25.0198, -15.9935) knots 0 0 0 1 2 2 2
  spline S132 degree 2 poles (25.0198, -15.9935) (25.0477, -16.5052) (25.6437, -17.3566) (26.2542, -17.7216) knots 0 0 0 1 2 2 2
  line L142 (24.3583, -20.7332) -> (24.9808, -19.9788)
  line L143 (24.9808, -19.9788) -> (25.88, -20.7208)
  line L144 (25.88, -20.7208) -> (25.2575, -21.4752)
  line L145 (25.2575, -21.4752) -> (24.3583, -20.7332)
  line L146 (21.7291, -18.5638) -> (22.3517, -17.8093)
  line L147 (22.3517, -17.8093) -> (23.2509, -18.5513)
  line L148 (23.2509, -18.5513) -> (22.6284, -19.3058)
  line L149 (22.6284, -19.3058) -> (21.7291, -18.5638)
  spline S133 degree 2 poles (20.9962, -26.8613) (21.1722, -26.7254) (21.4537, -26.3707) (21.5705, -26.1744) knots 0 0 0 1 2 2 2
  spline S134 degree 2 poles (21.5705, -26.1744) (21.6755, -25.9871) (21.7975, -25.6682) (21.8391, -25.5362) knots 0 0 0 1 2 2 2
  line L150 (21.8391, -25.5362) -> (21.8782, -25.506)
  line L151 (21.8782, -25.506) -> (22.4066, -26.1902)
  spline S135 degree 2 poles (22.4066, -26.1902) (22.2831, -26.4666) (21.7017, -27.209) (21.3772, -27.4597) knots 0 0 0 1 2 2 2
  spline S136 degree 2 poles (21.3772, -27.4597) (21.0488, -27.7133) (20.4574, -27.9579) (20.1493, -27.9711) knots 0 0 0 1 2 2 2
  spline S137 degree 2 poles (20.1493, -27.9711) (19.8204, -27.9817) (19.2603, -27.709) (19.0308, -27.4119) knots 0 0 0 1 2 2 2
  spline S138 degree 2 poles (19.0308, -27.4119) (18.7228, -27.0131) (18.7816, -26.0064) (19.0888, -25.6443) knots 0 0 0 1 2 2 2
  line L152 (19.0888, -25.6443) -> (19.0525, -25.5974)
  spline S139 degree 2 poles (19.0525, -25.5974) (18.8759, -25.6839) (18.4192, -25.8119) (18.1619, -25.7859) knots 0 0 0 1 2 2 2
  spline S140 degree 2 poles (18.1619, -25.7859) (17.9077, -25.7638) (17.3818, -25.4709) (17.1372, -25.1542) knots 0 0 0 1 2 2 2
  spline S141 degree 2 poles (17.1372, -25.1542) (16.8866, -24.8297) (16.6837, -24.1063) (16.7239, -23.7381) knots 0 0 0 1 2 2 2
  spline S142 degree 2 poles (16.7239, -23.7381) (16.7659, -23.3561) (17.189, -22.6674) (17.5682, -22.3745) knots 0 0 0 1 2 2 2
  spline S143 degree 2 poles (17.5682, -22.3745) (17.9318, -22.0936) (18.7793, -21.72) (19.1153, -21.654) knots 0 0 0 1 2 2 2
  line L153 (19.1153, -21.654) -> (19.6437, -22.3382)
  line L154 (19.6437, -22.3382) -> (19.5968, -22.3744)
  spline S144 degree 2 poles (19.5968, -22.3744) (19.2787, -22.3829) (18.3793, -22.6406) (18.0391, -22.9033) knots 0 0 0 1 2 2 2
  spline S145 degree 2 poles (18.0391, -22.9033) (17.8397, -23.0573) (17.5376, -23.4905) (17.5164, -23.7378) knots 0 0 0 1 2 2 2
  spline S146 degree 2 poles (17.5164, -23.7378) (17.4991, -23.9821) (17.628, -24.4318) (17.8303, -24.6938) knots 0 0 0 1 2 2 2
  spline S147 degree 2 poles (17.8303, -24.6938) (18.0326, -24.9557) (18.4478, -25.1781) (18.6601, -25.1702) knots 0 0 0 1 2 2 2
  spline S148 degree 2 poles (18.6601, -25.1702) (18.8724, -25.1622) (19.3012, -24.9496) (19.5202, -24.7805) knots 0 0 0 1 2 2 2
  line L155 (19.5202, -24.7805) -> (19.7939, -24.5692)
  line L156 (19.7939, -24.5692) -> (20.2076, -25.1048)
  line L157 (20.2076, -25.1048) -> (19.9925, -25.2709)
  spline S149 degree 2 poles (19.9925, -25.2709) (19.5585, -25.606) (19.3313, -26.4432) (19.6363, -26.8381) knots 0 0 0 1 2 2 2
  spline S150 degree 2 poles (19.6363, -26.8381) (19.7782, -27.0219) (20.1213, -27.1751) (20.295, -27.1657) knots 0 0 0 1 2 2 2
  spline S151 degree 2 poles (20.295, -27.1657) (20.4796, -27.1542) (20.8281, -26.9912) (20.9962, -26.8613) knots 0 0 0 1 2 2 2
  line L158 (14.1121, -24.8519) -> (14.9543, -24.3545)
  line L159 (14.9543, -24.3545) -> (15.5471, -25.3584)
  line L160 (15.5471, -25.3584) -> (14.7048, -25.8558)
  line L161 (14.7048, -25.8558) -> (14.1121, -24.8519)
  line L162 (9.6084, -26.9793) -> (13.0575, -25.4839)
  line L163 (13.0575, -25.4839) -> (13.4014, -26.277)
  spline S152 degree 2 poles (13.4014, -26.277) (13.181, -26.7872) (12.8003, -27.7222) (12.6344, -28.2088) knots 0 0 0 1 2 2 2
  spline S153 degree 2 poles (12.6344, -28.2088) (12.2999, -29.1883) (12.1986, -30.2338) (12.3931, -30.6825) knots 0 0 0 1 2 2 2
  spline S154 degree 2 poles (12.3931, -30.6825) (12.4953, -30.9182) (12.7936, -31.2088) (12.9742, -31.2651) knots 0 0 0 1 2 2 2
  spline S155 degree 2 poles (12.9742, -31.2651) (13.1548, -31.3214) (13.5483, -31.2854) (13.7568, -31.195) knots 0 0 0 1 2 2 2
  spline S156 degree 2 poles (13.7568, -31.195) (13.9563, -31.1085) (14.3209, -30.832) (14.4734, -30.6744) knots 0 0 0 1 2 2 2
  spline S157 degree 2 poles (14.4734, -30.6744) (14.6045, -30.5421) (14.8205, -30.2331) (14.8836, -30.1303) knots 0 0 0 1 2 2 2
  line L164 (14.8836, -30.1303) -> (14.9244, -30.1127)
  line L165 (14.9244, -30.1127) -> (15.2703, -30.9103)
  spline S158 degree 2 poles (15.2703, -30.9103) (15.0882, -31.1239) (14.3551, -31.7056) (13.9835, -31.8667) knots 0 0 0 1 2 2 2
  spline S159 degree 2 poles (13.9835, -31.8667) (13.1994, -32.2067) (11.9559, -31.7605) (11.6494, -31.0534) knots 0 0 0 1 2 2 2
  spline S160 degree 2 poles (11.6494, -31.0534) (11.5059, -30.7225) (11.4203, -30.1028) (11.4541, -29.8081) knots 0 0 0 1 2 2 2
  spline S161 degree 2 poles (11.4541, -29.8081) (11.4839, -29.5044) (11.6699, -28.8531) (11.7873, -28.5276) knots 0 0 0 1 2 2 2
  spline S162 degree 2 poles (11.7873, -28.5276) (11.9738, -27.989) (12.4818, -26.7888) (12.636, -26.4366) knots 0 0 0 1 2 2 2
  line L166 (12.636, -26.4366) -> (9.8894, -27.6274)
  line L167 (9.8894, -27.6274) -> (9.6084, -26.9793)
  spline S163 degree 2 poles (5.7346, -30.0249) (5.6261, -29.5989) (5.7137, -28.8017) (5.8944, -28.4702) knots 0 0 0 1 2 2 2
  spline S164 degree 2 poles (5.8944, -28.4702) (6.075, -28.1388) (6.7378, -27.6386) (7.1974, -27.5216) knots 0 0 0 1 2 2 2
  spline S165 degree 2 poles (7.1974, -27.5216) (7.6187, -27.4143) (8.4896, -27.3913) (8.829, -27.4629) knots 0 0 0 1 2 2 2
  line L168 (8.829, -27.4629) -> (9.0423, -28.3007)
  line L169 (9.0423, -28.3007) -> (8.9849, -28.3153)
  spline S166 degree 2 poles (8.9849, -28.3153) (8.8769, -28.2715) (8.4931, -28.1857) (8.2677, -28.1615) knots 0 0 0 1 2 2 2
  spline S167 degree 2 poles (8.2677, -28.1615) (8.0124, -28.1399) (7.6015, -28.1476) (7.3574, -28.2098) knots 0 0 0 1 2 2 2
  spline S168 degree 2 poles (7.3574, -28.2098) (7.118, -28.2708) (6.7119, -28.5577) (6.5967, -28.7859) knots 0 0 0 1 2 2 2
  spline S169 degree 2 poles (6.5967, -28.7859) (6.4934, -29.0008) (6.4596, -29.509) (6.5401, -29.8249) knots 0 0 0 1 2 2 2
  spline S170 degree 2 poles (6.5401, -29.8249) (6.6206, -30.1409) (6.8953, -30.4991) (7.0922, -30.5917) knots 0 0 0 1 2 2 2
  spline S171 degree 2 poles (7.0922, -30.5917) (7.2976, -30.6974) (7.8271, -30.6951) (8.1287, -30.6183) knots 0 0 0 1 2 2 2
  spline S172 degree 2 poles (8.1287, -30.6183) (8.4543, -30.5354) (9.0749, -30.2703) (9.2602, -30.1772) knots 0 0 0 1 2 2 2
  line L170 (9.2602, -30.1772) -> (10.0356, -33.2219)
  line L171 (10.0356, -33.2219) -> (6.7947, -34.0473)
  line L172 (6.7947, -34.0473) -> (6.6179, -33.3531)
  line L173 (6.6179, -33.3531) -> (9.0977, -32.7216)
  line L174 (9.0977, -32.7216) -> (8.6966, -31.1466)
  spline S173 degree 2 poles (8.6966, -31.1466) (8.5578, -31.2023) (8.2838, -31.2874) (8.1689, -31.3166) knots 0 0 0 1 2 2 2
  spline S174 degree 2 poles (8.1689, -31.3166) (7.7142, -31.4325) (7.0492, -31.4438) (6.7059, -31.2967) knots 0 0 0 1 2 2 2
  spline S175 degree 2 poles (6.7059, -31.2967) (6.3578, -31.1509) (5.8712, -30.5611) (5.7346, -30.0249) knots 0 0 0 1 2 2 2
  line L175 (4.1816, -34.6931) -> (4.0964, -32.3168)
  line L176 (4.0964, -32.3168) -> (4.6316, -32.2573)
  line L177 (4.6316, -32.2573) -> (5.0703, -34.5943)
  line L178 (5.0703, -34.5943) -> (4.1816, -34.6931)
  line L179 (2.6498, -34.8634) -> (2.5646, -32.487)
  line L180 (2.5646, -32.487) -> (3.0997, -32.4275)
  line L181 (3.0997, -32.4275) -> (3.5384, -34.7646)
  line L182 (3.5384, -34.7646) -> (2.6498, -34.8634)
  line L183 (-6.1343, -27.9964) -> (-5.3318, -28.1082)
  line L184 (-5.3318, -28.1082) -> (-5.7435, -31.0634)
  line L185 (-5.7435, -31.0634) -> (-2.9644, -31.4506)
  line L186 (-2.9644, -31.4506) -> (-2.5527, -28.4953)
  line L187 (-2.5527, -28.4953) -> (-1.7503, -28.6071)
  line L188 (-1.7503, -28.6071) -> (-2.5913, -34.6448)
  line L189 (-2.5913, -34.6448) -> (-3.3938, -34.533)
  line L190 (-3.3938, -34.533) -> (-3.0639, -32.1649)
  line L191 (-3.0639, -32.1649) -> (-5.843, -31.7778)
  line L192 (-5.843, -31.7778) -> (-6.1729, -34.1459)
  line L193 (-6.1729, -34.1459) -> (-6.9753, -34.0341)
  line L194 (-6.9753, -34.0341) -> (-6.1343, -27.9964)
  spline S176 degree 2 poles (-8.5585, -27.1753) (-7.9566, -27.3525) (-7.4811, -28.2391) (-7.7001, -28.9831) knots 0 0 0 1 2 2 2
  line L195 (-7.7001, -28.9831) -> (-8.4155, -31.4143)
  line L196 (-8.4155, -31.4143) -> (-7.9179, -31.5607)
  line L197 (-7.9179, -31.5607) -> (-8.0978, -32.172)
  line L198 (-8.0978, -32.172) -> (-8.5954, -32.0256)
  line L199 (-8.5954, -32.0256) -> (-8.9664, -33.2862)
  line L200 (-8.9664, -33.2862) -> (-9.7057, -33.0686)
  line L201 (-9.7057, -33.0686) -> (-9.3347, -31.808)
  line L202 (-9.3347, -31.808) -> (-10.6948, -31.4078)
  line L203 (-10.6948, -31.4078) -> (-10.5149, -30.7964)
  line L204 (-10.5149, -30.7964) -> (-9.1548, -31.1967)
  line L205 (-9.1548, -31.1967) -> (-8.5398, -29.1068)
  spline S177 degree 2 poles (-8.5398, -29.1068) (-8.4422, -28.775) (-8.3585, -28.4031) (-8.393, -28.223) knots 0 0 0 1 2 2 2
  spline S178 degree 2 poles (-8.393, -28.223) (-8.4189, -28.0661) (-8.677, -27.8408) (-8.9329, -27.7655) knots 0 0 0 1 2 2 2
  spline S179 degree 2 poles (-8.9329, -27.7655) (-9.113, -27.7125) (-9.4816, -27.7225) (-9.5672, -27.7333) knots 0 0 0 1 2 2 2
  line L206 (-9.5672, -27.7333) -> (-9.6098, -27.7208)
  line L207 (-9.6098, -27.7208) -> (-9.4146, -27.0573)
  spline S180 degree 2 poles (-9.4146, -27.0573) (-9.1893, -27.0618) (-8.7433, -27.121) (-8.5585, -27.1753) knots 0 0 0 1 2 2 2
  line L208 (-12.5262, -29.4328) -> (-11.6204, -29.802)
  line L209 (-11.6204, -29.802) -> (-12.0605, -30.8816)
  line L210 (-12.0605, -30.8816) -> (-12.9662, -30.5123)
  line L211 (-12.9662, -30.5123) -> (-12.5262, -29.4328)
  line L212 (-11.2395, -26.2763) -> (-10.3337, -26.6455)
  line L213 (-10.3337, -26.6455) -> (-10.7738, -27.7251)
  line L214 (-10.7738, -27.7251) -> (-11.6795, -27.3559)
  line L215 (-11.6795, -27.3559) -> (-11.2395, -26.2763)
  spline S181 degree 2 poles (-19.378, -28.0511) (-19.1959, -28.1785) (-18.7733, -28.3414) (-18.5511, -28.3944) knots 0 0 0 1 2 2 2
  spline S182 degree 2 poles (-18.5511, -28.3944) (-18.341, -28.4388) (-18.0003, -28.4601) (-17.8619, -28.4605) knots 0 0 0 1 2 2 2
  line L216 (-17.8619, -28.4605) -> (-17.8214, -28.4888)
  line L217 (-17.8214, -28.4888) -> (-18.3169, -29.1972)
  spline S183 degree 2 poles (-18.3169, -29.1972) (-18.6176, -29.1617) (-19.4996, -28.8282) (-19.8356, -28.5932) knots 0 0 0 1 2 2 2
  spline S184 degree 2 poles (-19.8356, -28.5932) (-20.1756, -28.3553) (-20.5854, -27.8638) (-20.6899, -27.5737) knots 0 0 0 1 2 2 2
  spline S185 degree 2 poles (-20.6899, -27.5737) (-20.7981, -27.2629) (-20.7048, -26.6469) (-20.4896, -26.3392) knots 0 0 0 1 2 2 2
  spline S186 degree 2 poles (-20.4896, -26.3392) (-20.2008, -25.9263) (-19.2224, -25.6823) (-18.7852, -25.8675) knots 0 0 0 1 2 2 2
  line L218 (-18.7852, -25.8675) -> (-18.7512, -25.8189)
  spline S187 degree 2 poles (-18.7512, -25.8189) (-18.8865, -25.6761) (-19.1448, -25.2784) (-19.1967, -25.0251) knots 0 0 0 1 2 2 2
  spline S188 degree 2 poles (-19.1967, -25.0251) (-19.2515, -24.7758) (-19.1287, -24.1865) (-18.8993, -23.8586) knots 0 0 0 1 2 2 2
  spline S189 degree 2 poles (-18.8993, -23.8586) (-18.6643, -23.5226) (-18.0344, -23.1132) (-17.671, -23.0418) knots 0 0 0 1 2 2 2
  spline S190 degree 2 poles (-17.671, -23.0418) (-17.2938, -22.968) (-16.5102, -23.1664) (-16.1176, -23.441) knots 0 0 0 1 2 2 2
  spline S191 degree 2 poles (-16.1176, -23.441) (-15.7411, -23.7044) (-15.1317, -24.4018) (-14.9685, -24.7029) knots 0 0 0 1 2 2 2
  line L219 (-14.9685, -24.7029) -> (-15.464, -25.4113)
  line L220 (-15.464, -25.4113) -> (-15.5126, -25.3773)
  spline S192 degree 2 poles (-15.5126, -25.3773) (-15.6155, -25.0762) (-16.1298, -24.2946) (-16.482, -24.0482) knots 0 0 0 1 2 2 2
  spline S193 degree 2 poles (-16.482, -24.0482) (-16.6884, -23.9038) (-17.1919, -23.7446) (-17.4343, -23.7981) knots 0 0 0 1 2 2 2
  spline S194 degree 2 poles (-17.4343, -23.7981) (-17.6727, -23.8545) (-18.0635, -24.1116) (-18.2532, -24.3828) knots 0 0 0 1 2 2 2
  spline S195 degree 2 poles (-18.2532, -24.3828) (-18.4429, -24.6541) (-18.5314, -25.1167) (-18.4605, -25.317) knots 0 0 0 1 2 2 2
  spline S196 degree 2 poles (-18.4605, -25.317) (-18.3896, -25.5173) (-18.0588, -25.8632) (-17.8321, -26.0217) knots 0 0 0 1 2 2 2
  line L221 (-17.8321, -26.0217) -> (-17.5487, -26.2199)
  line L222 (-17.5487, -26.2199) -> (-17.9366, -26.7745)
  line L223 (-17.9366, -26.7745) -> (-18.1592, -26.6188)
  spline S197 degree 2 poles (-18.1592, -26.6188) (-18.6086, -26.3045) (-19.4755, -26.3372) (-19.7614, -26.7461) knots 0 0 0 1 2 2 2
  spline S198 degree 2 poles (-19.7614, -26.7461) (-19.8945, -26.9363) (-19.9385, -27.3095) (-19.8777, -27.4726) knots 0 0 0 1 2 2 2
  spline S199 degree 2 poles (-19.8777, -27.4726) (-19.8116, -27.6454) (-19.5521, -27.9293) (-19.378, -28.0511) knots 0 0 0 1 2 2 2
  line L224 (-19.5129, -20.8809) -> (-18.787, -21.5365)
  line L225 (-18.787, -21.5365) -> (-19.5685, -22.4017)
  line L226 (-19.5685, -22.4017) -> (-20.2943, -21.7461)
  line L227 (-20.2943, -21.7461) -> (-19.5129, -20.8809)
  spline S200 degree 2 poles (-25.2168, -19.1816) (-23.9751, -18.1101) (-22.1891, -17.8283) (-21.5404, -18.5801) knots 0 0 0 1 2 2 2
  spline S201 degree 2 poles (-21.5404, -18.5801) (-20.882, -19.3431) (-21.4512, -21.0805) (-22.6668, -22.1293) knots 0 0 0 1 2 2 2
  spline S202 degree 2 poles (-22.6668, -22.1293) (-23.916, -23.2072) (-25.6946, -23.4826) (-26.3465, -22.7271) knots 0 0 0 1 2 2 2
  spline S203 degree 2 poles (-26.3465, -22.7271) (-27.0016, -21.9679) (-26.4212, -20.2208) (-25.2168, -19.1816) knots 0 0 0 1 2 2 2
  spline S204 degree 2 poles (-23.1264, -18.761) (-23.432, -18.8681) (-24.1997, -19.4001) (-24.6747, -19.8099) knots 0 0 0 1 2 2 2
  spline S205 degree 2 poles (-24.6747, -19.8099) (-25.1497, -20.2198) (-25.7845, -20.8981) (-25.9395, -21.1949) knots 0 0 0 1 2 2 2
  spline S206 degree 2 poles (-25.9395, -21.1949) (-26.0944, -21.4917) (-26.0567, -22.0269) (-25.8341, -22.285) knots 0 0 0 1 2 2 2
  spline S207 degree 2 poles (-25.8341, -22.285) (-25.6114, -22.543) (-25.081, -22.6661) (-24.754, -22.5536) knots 0 0 0 1 2 2 2
  spline S208 degree 2 poles (-24.754, -22.5536) (-24.4377, -22.4438) (-23.6615, -21.8915) (-23.209, -21.501) knots 0 0 0 1 2 2 2
  spline S209 degree 2 poles (-23.209, -21.501) (-22.7227, -21.0814) (-22.1236, -20.4601) (-21.9532, -20.1434) knots 0 0 0 1 2 2 2
  spline S210 degree 2 poles (-21.9532, -20.1434) (-21.7913, -19.847) (-21.8204, -19.2915) (-22.0528, -19.0222) knots 0 0 0 1 2 2 2
  spline S211 degree 2 poles (-22.0528, -19.0222) (-22.2722, -18.7679) (-22.8026, -18.6448) (-23.1264, -18.761) knots 0 0 0 1 2 2 2
  line L228 (-30.0173, -17.9286) -> (-27.9287, -16.792)
  line L229 (-27.9287, -16.792) -> (-27.6367, -17.2444)
  line L230 (-27.6367, -17.2444) -> (-29.5324, -18.6798)
  line L231 (-29.5324, -18.6798) -> (-30.0173, -17.9286)
  line L232 (-29.1814, -19.2235) -> (-27.0928, -18.0869)
  line L233 (-27.0928, -18.0869) -> (-26.8007, -18.5393)
  line L234 (-26.8007, -18.5393) -> (-28.6964, -19.9747)
  line L235 (-28.6964, -19.9747) -> (-29.1814, -19.2235)
  dimension "d142" = 57.15
  constraints: 1 centre point, 1 coincident, 1 other
  measures "d142" diameter of A0
extrude "Extrusion18" cut sketch "Sketch24" against normal blind 1.27